Autodesk Inventor part; units mm, degrees
(part 2 of 2)
sketch "Эскиз16" plane through (8.25, 13, 36.2214) normal (0, 0, -1) x (-1, 0, 0)
  line L0 (0, 0) -> (0, 4.5) projected
  line L1 (0, 4.5) -> (0, 8)
  line L2 (0, 8) -> (1, 8)
  line L3 (0, 4.5) -> (-4.75, 4.5) projected
  line L4 (0, 4.5) -> (3, 4.5)
  line L5 (14.25, 4.5) -> (2.25, 4.5) projected
  line L6 (1, 8) -> (3, 4.5)
  line L7 (8.25, 4.5) -> (8.25, 0) construction
  line L8 (14.25, 0) -> (2.25, 0) construction
  line L9 (16.5, 4.5) -> (16.5, 8)
  line L10 (16.5, 8) -> (15.5, 8)
  line L11 (16.5, 4.5) -> (13.5, 4.5)
  line L12 (15.5, 8) -> (13.5, 4.5)
  point P0 (8.25, -13)
  dimension "d201" = 3.5
  dimension "d202" = 1
  dimension "d203" = 3
  constraints: 18 end point, 4 symmetric about line, 2 midpoint, 1 perpendicular, 1 point on line, 1 vertical
  measures "d201" distance of L0.end L1.end
  measures "d202" distance of L1.end L2.end
  measures "d203" distance of L0.end L4.end
extrude "Выдавливание14" add sketch "Эскиз16" against normal blind 25.5
extrude "Выдавливание15" add sketch "Эскиз14" along normal blind 4.5 contours L6 A1 L24 A0 | A0 L24 L14 L13 | L23 A1 L5 A0 | A0 L12 L14 L23
